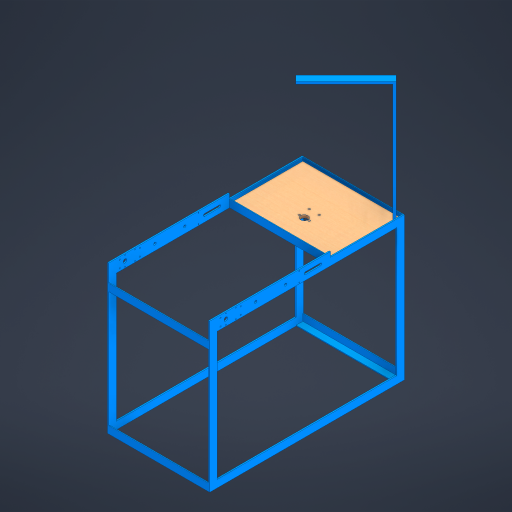
# Autodesk Inventor part: Structure
Saved by Autodesk Inventor 2023 (Build 270158000, 158)
## iProperties
Created: 2023-11-03
Part Number: Structure
Material: Generic
Document SubType Name: Modeling
Designer: Abhinav
Density: 1 g/cm^3
Appearance: Default(1)
Author: Abhinav
Autodesk Inventor part; units mm, degrees
ref_plane "YZ Plane" through (0, 0, 0) normal (1, 0, 0) x (0, 1, 0)
ref_plane "XZ Plane" through (0, 0, 0) normal (0, 1, 0) x (-1, 0, 0)
ref_plane "XY Plane" through (0, 0, 0) normal (0, 0, 1) x (1, 0, 0)
sketch "Sketch1" plane through (0, 0, 0) normal (1, 0, 0) x (0, 1, 0)
  line L0 (0, -410) -> (0, 0)
  line L1 (-25, 0) -> (-25, -25) construction
  circle A0 centre (-25, -25) radius 5.1
  circle A1 centre (-25, -145) radius 5.1
  circle A2 centre (-25, -265) radius 5.1
  circle A3 centre (-25, -385) radius 5.1 construction
  line L2 (0, -420) -> (0, -410)
  line L3 (-50, -35) -> (-50, 0)
  line L4 (-55.25, -1) -> (-55.25, -91.5825) construction
  arc A4 (-55.25, -91.5825) -> (5.25, -91.5825) centre (-25, -1) ccw construction
  line L5 (5.25, -91.5825) -> (5.25, -1) construction
  line L6 (5.25, -1) -> (-55.25, -1) construction
  circle A5 centre (-5, -65) radius 2
  circle A6 centre (-45, -65) radius 2
  circle A7 centre (-45, -25) radius 2
  circle A8 centre (-5, -25) radius 2
  circle A9 centre (-25, -25) radius 7.5
  line L7 (0, 435) -> (0, 0) construction
  line L8 (-50, 432) -> (-50, 405) construction
  line L9 (-50, -5) -> (-50, -125) construction
  line L10 (-25, -25) -> (-5, -25) construction
  circle A10 centre (-40, -84.5) radius 2.5
  line L11 (-40, -84.5) -> (-10, -84.5) construction
  circle A11 centre (-40, -84.5) radius 2.5
  circle A12 centre (-10, -84.5) radius 2.5
  circle A13 centre (-40, -3.5) radius 2.5
  circle A14 centre (-10, -3.5) radius 2.5
  line L12 (-40, -3.5) -> (-10, -3.5) construction
  circle A15 centre (-25, -25) radius 3.9303 construction
  line L13 (-10, -3.5) -> (-40, -84.5) construction
  line L14 (-25, -4) -> (-25, -3.5) construction
  line L15 (-15, 435) -> (-15, 405) construction
  circle A16 centre (-15, 405) radius 4 construction
  circle A17 centre (-15, 373) radius 4 construction
  circle A18 centre (-15, 341) radius 4 construction
  circle A19 centre (-15, 309) radius 4 construction
  circle A20 centre (-15, 277) radius 4 construction
  circle A21 centre (-15, 245) radius 4 construction
  circle A22 centre (-25, -375) radius 4 construction
  line L16 (-25, -375) -> (-25, -405) construction
  line L17 (-25, -375) -> (-25, -345) construction
  line L18 (-25, -405) -> (-25, -345) construction
  line L19 (-30.1, -405) -> (-30.1, -345)
  line L20 (-19.9, -345) -> (-19.9, -405)
  arc A23 (-30.1, -405) -> (-19.9, -405) centre (-25, -405) ccw
  arc A24 (-19.9, -345) -> (-30.1, -345) centre (-25, -345) ccw
  line L21 (-25, -405) -> (-25, -445) construction
  line L22 (0, -420) -> (0, -445)
  line L23 (-25, -375) -> (-25, -320) construction
  line L24 (-25, -320) -> (-5, -320) construction
  circle A25 centre (-5, -320) radius 2
  circle A26 centre (-45, -320) radius 2
  line L25 (-50, 435) -> (-595, 435) construction
  line L26 (-595, 435) -> (-595, 405) construction
  line L27 (-565, 405) -> (-50, 405) construction
  line L28 (-50, 405) -> (-50, 432) construction
  line L29 (-45, -742) -> (-595, -742)
  line L30 (-595, -742) -> (-595, -712)
  line L31 (-565, -712) -> (-50, -712)
  line L32 (-595, -712) -> (-565, -712) construction
  line L33 (-595, 405) -> (-595, -742)
  line L34 (-50, 0) -> (-120.4948, 0)
  line L35 (-50, -390) -> (-50, -225) construction
  line L36 (-50, -195) -> (-50, -225)
  line L37 (-50, -390) -> (-50, -420)
  line L38 (-50, -445) -> (-50, -420)
  line L39 (-50, -445) -> (-50, -742)
  line L40 (-565, -742) -> (-565, -225)
  line L41 (-50, -35) -> (-50, -195)
  line L42 (-50, -225) -> (-50, -390)
  line L43 (-50, 435) -> (0, 435) construction
  line L44 (0, 435) -> (0, 432) construction
  line L45 (0, 432) -> (-50, 432) construction
  line L46 (-50, 432) -> (-50, 435) construction
  line L47 (-565, -742) -> (-595, -742)
  line L48 (-595, -742) -> (-595, -739)
  line L49 (-592, -739) -> (-565, -739)
  line L50 (-565, -739) -> (-565, -742)
  line L51 (-595, -742) -> (-592, -742)
  line L52 (-592, -739) -> (-592, -712)
  line L53 (-595, -712) -> (-595, -742)
  line L54 (-595, 435) -> (-565, 435) construction
  line L55 (-565, 435) -> (-565, 432) construction
  line L56 (-565, 432) -> (-592, 432) construction
  line L57 (-595, 432) -> (-595, 435) construction
  line L58 (-595, 435) -> (-592, 435) construction
  line L59 (-592, 432) -> (-592, 405) construction
  line L60 (-592, 405) -> (-595, 405) construction
  line L61 (-595, 405) -> (-595, 435) construction
  line L62 (-595, -195) -> (-595, -225)
  line L63 (0, 0) -> (0, 10)
  line L64 (-50, 10) -> (-565, 10)
  line L65 (-565, 10) -> (-565, 40) construction
  line L66 (-565, 40) -> (0, 40)
  line L67 (0, 40) -> (0, 10)
  line L68 (-565, 40) -> (-595, 40)
  line L69 (-565, -195) -> (-565, 10)
  line L70 (-565, 40) -> (-565, 405) construction
  line L71 (-565, -225) -> (-565, -195)
  line L72 (-595, 40) -> (-592, 40)
  line L73 (-592, 37) -> (-592, 10)
  line L74 (-592, 10) -> (-595, 10)
  line L75 (-595, 10) -> (-595, 40)
  line L76 (-595, 40) -> (-565, 40)
  line L77 (-565, 40) -> (-565, 37)
  line L78 (-565, 37) -> (-592, 37)
  line L79 (-595, 37) -> (-595, 40)
  line L80 (0, 432) -> (-50, 432) construction
  line L81 (-50, 432) -> (-50, 435) construction
  line L82 (-50, 435) -> (0, 435) construction
  line L83 (0, 435) -> (0, 432) construction
  line L84 (-50, -5) -> (-50, 10)
  line L85 (-50, 40) -> (-50, 405) construction
  line L86 (0, -445) -> (-50, -445)
  line L87 (-50, -445) -> (-20, -445)
  line L88 (-20, -445) -> (-20, -448)
  line L89 (-20, -448) -> (-47, -448)
  line L90 (-50, -448) -> (-50, -445)
  line L91 (-50, -445) -> (-47, -445)
  line L92 (-47, -448) -> (-47, -475)
  line L93 (-47, -475) -> (-50, -475)
  line L94 (-50, -475) -> (-50, -445)
  line L95 (-50, -445) -> (-20, -445)
  line L96 (-20, -445) -> (-20, -742)
  line L97 (-20, -742) -> (-50, -742)
  line L98 (-50, -742) -> (-50, -445)
  line L99 (-20, -742) -> (-50, -742)
  line L100 (-50, -742) -> (-50, -739)
  line L101 (-47, -739) -> (-20, -739)
  line L102 (-20, -739) -> (-20, -742)
  line L103 (-50, -712) -> (-47, -712)
  line L104 (-47, -712) -> (-47, -739)
  line L105 (-47, -742) -> (-50, -742)
  line L106 (-50, -742) -> (-50, -712)
  line L107 (-592, -712) -> (-595, -712)
  line L108 (-50, 40) -> (-70, 40) construction
  line L109 (-70, 40) -> (-100, 40)
  line L110 (-100, 40) -> (-100, 37)
  line L111 (-100, 37) -> (-70, 37)
  line L112 (-70, 37) -> (-70, 40)
  point P0 (0, -93.1697)
  point P1 (0, -1)
  point P2 (-54.9, 0)
  point P3 (0, 40)
  point P4 (-50, -742)
  point P5 (-50, -712)
  point P6 (-50, -712)
  dimension "d12" = 25
  dimension "d13" = 10.2
  dimension "d16" = 120
  dimension "d30" = 4
  dimension "d96" = 30
  dimension "d114" = 30
  dimension "d115" = 0.5
  dimension "d116" = 30
  dimension "d117" = 8
  dimension "d120" = 32
  dimension "d151" = 30
  dimension "d152" = 30
  dimension "d153" = 40
  dimension "d155" = 55
  dimension "d156" = 20
  dimension "d157" = 4
  dimension "d159" = 30
  dimension "d160" = 30
  dimension "d161" = 30
  dimension "d162" = 165
  dimension "d164" = 3
  dimension "d165" = 3
  dimension "d167" = 3
  dimension "d168" = 3
  dimension "d173" = 30
  dimension "d174" = 3
  dimension "d175" = 30
  dimension "d176" = 3
  dimension "d177" = 30
  dimension "d183" = 30
  dimension "d186" = 20
  dimension "d187" = 30
  constraints: 228 end point, 37 parallel, 27 centre point, 21 horizontal, 20 perpendicular, 13 point on line, 13 vertical, 8 coincident, 7 point on circle, 5 equal radius, 4 tangent, 2 collinear, 1 midpoint, 1 symmetric about line, 17 other
  measures "d12" distance of L1.start L1.end
  measures "d13" diameter of A0
  measures "d16" distance of A0.centre A1.centre
  measures "d30" diameter of A5
  measures "d96" distance of L8.end L25.start
  measures "d114" distance of L11.end L11.start
  measures "d115" distance of L14.start L14.end
  measures "d116" distance of L15.start L15.end
  measures "d117" diameter of A16
  measures "d120" distance of A16.centre A17.centre
  measures "d151" distance of L16.start L16.end
  measures "d152" distance of L16.start L17.end
  measures "d153" distance of L16.end L21.end
  measures "d155" distance of L23.start L23.end
  measures "d156" distance of L23.end L24.end
  measures "d157" diameter of A25
  measures "d159" distance of L26.end L25.end
  measures "d160" distance of L29.end L30.end
  measures "d161" distance of L27.start L33.start
  measures "d162" distance of L35.start L35.end
  measures "d164" distance of L7.start L44.end
  measures "d165" distance of L29.end L48.end
  measures "d167" distance of L54.end L55.end
  measures "d168" distance of L59.end L60.end
  measures "d173" distance of L64.end L65.end
  measures "d174" distance of L76.end L77.end
  measures "d175" distance of L88.end L90.start
  measures "d176" distance of L87.end L88.end
  measures "d177" distance of L91.end L92.end
  measures "d183" distance of L96.end L39.end
  measures "d186" distance of L85.start L108.end
  measures "d187" distance of L111.end L110.end
extrude "Extrusion1" add sketch "Sketch1" along normal blind 5 contours L2 L22 L86 L38 L37 L42 L36 L41 L3 L84 L64 L69 L71 L40 L49 L52 L107 L33 L74 L73 L78 L77 L66 L110 L111 L112 L67 L63 L0 | L88 L89 L92 L93 L39 L86 | L112 L111 L110 L66 | L96 L101 L104 L103 L39 L93 L92 L89 | L96 L97 L29 L39 L103 L104 L101 | L77 L78 L73 L74 L33 L68 | L39 L29 L40 L31 | L40 L29 L30 L107 L52 L49
ref_plane "Work Plane1" through (-200, 0, 0) normal (-1, 0, 0) x (0, 0, 1)
mirror "Mirror1" about plane through (-200, 0, 0) normal (-1, 0, 0) of "Extrusion1"
extrude "Extrusion4" add sketch "Sketch1" against normal up to next contours L88 L89 L92 L93 L39 L86 | L112 L111 L110 L66 | L96 L97 L29 L39 L103 L104 L101 | L77 L78 L73 L74 L33 L68 | L40 L29 L30 L107 L52 L49
sketch "Sketch5" plane through (0, -47, -25) normal (0, 1, 0) x (1, 0, 0)
  line L0 (-200, 520) -> (-200, 501) construction
  line L1 (0, 420) -> (0, -25) construction
  line L2 (0, 714) -> (-14.1421, 699.8579) construction
  line L3 (-1.7678, 691.019) -> (-22.981, 712.2322)
  line L4 (-22.981, 712.2322) -> (-26.5165, 708.6967)
  line L5 (-26.5165, 708.6967) -> (-5.3033, 687.4835)
  line L6 (-5.3033, 687.4835) -> (-1.7678, 691.019)
  line L7 (-1.7678, 691.019) -> (-26.5165, 708.6967) construction
  line L8 (-22.981, 712.2322) -> (-5.3033, 687.4835) construction
  line L9 (-26.5165, 708.6967) -> (-30.052, 705.1612)
  line L10 (-30.052, 705.1612) -> (-8.8388, 683.948)
  line L11 (-8.8388, 683.948) -> (-5.3033, 687.4835)
  line L12 (-405, 687) -> (-405, -35) projected
  line L13 (-200, 423) -> (-200, 520) construction
  line L14 (-169.75, 496) -> (-169.75, 586.5825) construction
  arc A0 (-169.75, 586.5825) -> (-230.25, 586.5825) centre (-200, 496) ccw construction
  line L15 (-230.25, 586.5825) -> (-230.25, 496) construction
  line L16 (-230.25, 496) -> (-169.75, 496) construction
  circle A1 centre (-220, 560) radius 4
  circle A2 centre (-180, 560) radius 4
  circle A3 centre (-180, 520) radius 4
  circle A4 centre (-220, 520) radius 4
  circle A5 centre (-200, 520) radius 15
  line L17 (0, 450) -> (0, 423) projected
  line L18 (0, 714) -> (-400, 714) projected
  line L19 (0, 423) -> (-400, 423)
  line L20 (-400, 423) -> (-400, 714)
  line L21 (-400, 714) -> (0, 714)
  line L22 (0, 714) -> (0, 423)
  point P0 (0, -25)
  point P1 (0, 420)
  point P2 (5, 423)
  point P3 (-405, 423)
  point P4 (0, 714)
  dimension "d144" = 20
  dimension "d145" = 30
  dimension "d146" = 5
  dimension "d150" = 5
  dimension "d178" = 97
  dimension "d182" = 30
  constraints: 38 end point, 6 centre point, 5 perpendicular, 4 parallel, 2 midpoint, 2 point on circle, 1 horizontal, 1 point on line, 2 other
  measures "d144" distance of L2.start L2.end
  measures "d145" distance of L3.start L3.end
  measures "d146" distance of L4.end L3.end
  measures "d150" distance of L4.end L9.end
  measures "d178" distance of L13.start L13.end
  measures "d182" diameter of A5
extrude "Extrusion6" add sketch "Sketch5" along normal blind 12 contours L6 L5 L4 L3 | L11 L10 L9 L5 | L17 L19 L20 L18 L22
extrude "Extrusion8" add sketch "Sketch5" along normal blind 500 contours L6 L5 L4 L3 | L11 L10 L9 L5
sketch "Sketch10" plane through (-8.8388, -47, -708.948) normal (-0.7071068, 0, 0.7071068) x (0.7071068, 0, 0.7071068)
  line L0 (0, 0) -> (0, 345) projected
  line L1 (-30, 500) -> (0, 500)
  line L2 (0, 500) -> (0, 490)
  line L3 (0, 490) -> (-30, 490)
  line L4 (-30, 490) -> (-30, 500)
  point P0 (507.5519, 47)
  dimension "d147" = 10
  constraints: 8 end point, 2 parallel, 1 horizontal, 1 perpendicular, 1 point on line
  measures "d147" distance of L1.end L2.end
extrude "Extrusion11" add sketch "Sketch10" along normal blind 275
body "Solid1"
